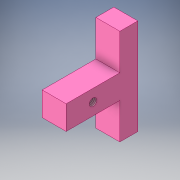
# Autodesk Inventor part: vexSupportForArm
Saved by Autodesk Inventor 2016 SP1 (Build 200210100, 210)
## iProperties
Created: 2015-07-13
Part Number: vexSupportForArm
Material: Aluminum 6061
Document SubType Name: Modeling
Designer: steele
Density: 2.7 g/cm^3
Appearance: Pink
Mass: 94.7579 g
Surface Area: 105.47 cm^2
Volume: 35.0955 cm^3
Author: steele
Autodesk Inventor part; units mm, degrees
ref_plane "YZ Plane" through (0, 0, 0) normal (1, 0, 0) x (0, 1, 0)
ref_plane "XZ Plane" through (0, 0, 0) normal (0, 1, 0) x (-1, 0, 0)
ref_plane "XY Plane" through (0, 0, 0) normal (0, 0, 1) x (1, 0, 0)
sketch "Sketch1" plane through (0, 0, 0) normal (0, 0, 1) x (1, 0, 0)
  line L0 (-6.35, -25.4) -> (6.35, -25.4)
  line L1 (6.35, -25.4) -> (6.35, 25.4)
  line L2 (6.35, 25.4) -> (-6.35, 25.4)
  line L3 (-6.35, 25.4) -> (-6.35, -25.4)
  line L4 (-6.35, -25.4) -> (6.35, 25.4) construction
  line L5 (6.35, -25.4) -> (-6.35, 25.4) construction
  point P0 (0, 0)
  dimension "height" = 50.8
  dimension "width" = 12.7
  constraints: 12 end point, 2 midpoint, 2 parallel, 1 horizontal, 1 perpendicular
  measures "height" distance of L0.end L1.end
  measures "width" distance of L1.end L2.end
extrude "Extrusion9" add sketch "Sketch1" against normal blind 9.525
sketch "Sketch19" plane through (0, 0, 0) normal (0, 0, 1) x (1, 0, 0)
  line L0 (-6.35, -6.35) -> (6.35, -6.35)
  line L1 (6.35, -6.35) -> (6.35, 6.35)
  line L2 (6.35, 6.35) -> (-6.35, 6.35)
  line L3 (-6.35, 6.35) -> (-6.35, -6.35)
  line L4 (-6.35, -6.35) -> (6.35, 6.35) construction
  line L5 (6.35, -6.35) -> (-6.35, 6.35) construction
  line L6 (-6.35, 25.4) -> (-6.35, -25.4) projected
  point P0 (0, 0)
  dimension "d126" = 12.7
  constraints: 12 end point, 2 midpoint, 2 parallel, 1 collinear, 1 perpendicular
  measures "d126" distance of L2.end L0.start
extrude "Extrusion10" add sketch "Sketch19" along normal blind 28.448
sketch "Sketch20" plane through (6.35, -25.4, -9.525) normal (1, 0, 0) x (0, 0, -1)
  line L0 (-9.525, 31.75) -> (-9.525, 50.8) projected
  point P0 (-9.525, 25.4)
  point P1 (-23.749, 25.4)
  dimension "d129" = 14.224
  measures "d129" distance from line of point (-23.749, 25.4) L0
hole "Hole13" at (6.35, 0, 14.224) direction (-1, 0, 0) diameter 3.9624 end through all thread size "10-32 UNF" class "2B" standard "ANSI Unified Screw Threads"
equation "\"height\" = partHeight"
equation "\"width\" = partWidth"
equation "\"d124\" = depthBehindPlate"
equation "\"d126\" = slotWidth"
equation "\"d127\" = 2 * centerLineOfCylinder"
equation "\"d129\" = centerLineOfCylinder"
equation "\"partWidth\" = 12.7"
equation "\"centerLineOfCylinder\" = 14.224"
equation "\"partHeight\" = 50.8"
equation "\"depthBehindPlate\" = 9.525"
equation "\"slotWidth\" = 12.7"
body "Solid2"
